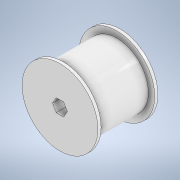
# Autodesk Inventor part: Polybelt Wheels
Saved by Autodesk Inventor 2022 (Build 260153000, 153)
## iProperties
Created: 2020-01-25
Part Number: Polybelt Wheels
Material: ABS Plastic
Document SubType Name: Modeling
Designer: aidan
Density: 1.06 g/cm^3
Appearance: White
Author: aidan
Autodesk Inventor part; units mm, degrees
ref_plane "YZ Plane" through (0, 0, 0) normal (1, 0, 0) x (0, 1, 0)
ref_plane "XZ Plane" through (0, 0, 0) normal (0, 1, 0) x (-1, 0, 0)
ref_plane "XY Plane" through (0, 0, 0) normal (0, 0, 1) x (1, 0, 0)
sketch "Sketch1" plane through (0, 0, 0) normal (0, 1, 0) x (-1, 0, 0)
  line L0 (31.75, -26.9875) -> (0, -26.9875)
  line L1 (0, -26.9875) -> (0, 26.9875)
  line L2 (0, 26.9875) -> (31.75, 26.9875)
  line L3 (31.75, 26.9875) -> (31.75, -26.9875)
  line L4 (0, -26.9875) -> (38.1, -26.9875)
  line L5 (38.1, -26.9875) -> (38.1, -30.1625)
  line L6 (38.1, -30.1625) -> (0, -30.1625)
  line L7 (0, -30.1625) -> (0, -26.9875)
  line L8 (0, 26.9875) -> (38.1, 26.9875)
  line L9 (38.1, 26.9875) -> (38.1, 30.1625)
  line L10 (38.1, 30.1625) -> (0, 30.1625)
  line L11 (0, 30.1625) -> (0, 26.9875)
  line L12 (0, 0) -> (51.6774, 0) construction
  point P0 (31.75, -26.9875)
  point P1 (31.75, 26.9875)
  dimension "d0" = 53.975
  dimension "d1" = 6.35
  dimension "d2" = 60.325
  dimension "d4" = 31.75
  constraints: 26 end point, 6 parallel, 4 horizontal, 3 perpendicular, 1 collinear, 1 midpoint, 2 other
  measures "d0" distance between parallel lines of L2 L0
  measures "d1" distance between parallel lines of L5 L3
  measures "d2" distance between parallel lines of L10 L6
  measures "d4" distance between parallel lines of L1 L3
revolve "Revolution1" add sketch "Sketch1" angle 360 about axis through (0, 0, -26.9875) along (0, 0, 1)
sketch "Sketch2" plane through (0, 0, 30.1625) normal (0, 0, 1) x (1, 0, 0)
  line L0 (7.479, 0) -> (3.7395, -6.477)
  line L1 (3.7395, -6.477) -> (-3.7395, -6.477)
  line L2 (-3.7395, -6.477) -> (-7.479, 0)
  line L3 (-7.479, 0) -> (-3.7395, 6.477)
  line L4 (-3.7395, 6.477) -> (3.7395, 6.477)
  line L5 (3.7395, 6.477) -> (7.479, 0)
  point P0 (0, 0)
  point P1 (0, 0)
  point P2 (0, 6.477)
  dimension "d6" = 12.954
  constraints: 12 end point, 1 coincident, 1 horizontal, 1 midpoint, 13 other
  measures "d6" distance between parallel lines of L1 L4
extrude "Extrusion1" cut sketch "Sketch2" against normal through all
equation "\"d4\" = d9"
equation "\"d9\" = 31.75"
body "Solid1"
